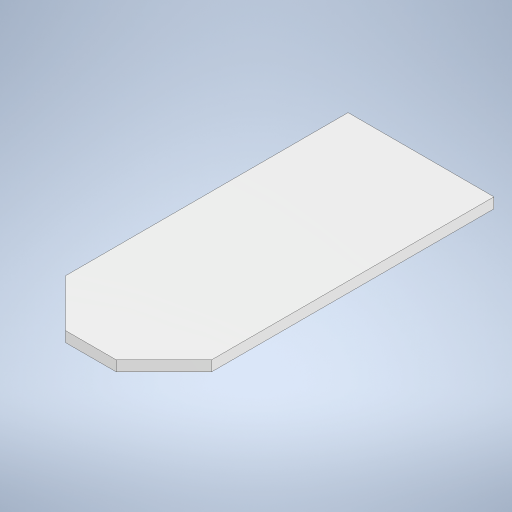
# Autodesk Inventor part: LightPad
Saved by Autodesk Inventor 2024 (Build 280153000, 153)
## iProperties
Created: 2023-11-03
Part Number: LightPad
Material: Acetal Resin, White
Document SubType Name: Modeling
Designer: njspada
Density: 1.425 g/cm^3
Appearance: Smooth - White
Author: njspada
Autodesk Inventor part; units mm, degrees
ref_plane "YZ Plane" through (0, 0, 0) normal (1, 0, 0) x (0, 1, 0)
ref_plane "XZ Plane" through (0, 0, 0) normal (0, 1, 0) x (-1, 0, 0)
ref_plane "XY Plane" through (0, 0, 0) normal (0, 0, 1) x (1, 0, 0)
sketch "Sketch1" plane through (0, 0, 0) normal (0, 1, 0) x (-1, 0, 0)
  line L0 (0, 0) -> (45.1612, 0)
  line L1 (45.1612, 0) -> (45.1612, -102.1842)
  line L2 (45.1612, -102.1842) -> (0, -102.1842)
  line L3 (0, -102.1842) -> (0, 0)
  line L4 (45.1612, 0) -> (45.1612, -14.732) construction
  line L5 (45.1612, -14.732) -> (0, -14.732) construction
  line L6 (45.1612, -14.732) -> (30.4292, 0)
  line L7 (45.1612, -14.732) -> (65.9954, -14.732) construction
  line L8 (0, -14.732) -> (14.732, 0)
  dimension "d0" = 45.1612
  dimension "d1" = 102.1842
  dimension "d2" = 14.732
  dimension "d3" = 135
  constraints: 18 end point, 4 point on line, 2 horizontal, 2 parallel, 2 perpendicular, 1 equal length
  measures "d0" distance of L1.end L2.end
  measures "d1" distance of L0.end L1.end
  measures "d2" distance of L0.end L4.end
  measures "d3" angle of L7 L6
extrude "Extrusion1" add sketch "Sketch1" along normal blind 3.2258 contours L0 L6 L1 L2 L3 L8
body "Solid1"
